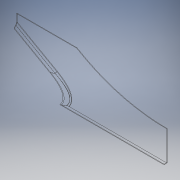
# Autodesk Inventor part: endplate
Saved by Autodesk Inventor 2018.2 (Build 222227000, 227)
## iProperties
Created: 2018-02-26
Part Number: endplate
Material: GFRC
Document SubType Name: Modeling
Designer: ku_sk
Density: 1.7 g/cm^3
Appearance: フラット - 研磨 グレー
Author: ku_sk
Autodesk Inventor part; units mm, degrees
ref_plane "YZ Plane" through (0, 0, 0) normal (1, 0, 0) x (0, 1, 0)
ref_plane "XZ Plane" through (0, 0, 0) normal (0, 1, 0) x (-1, 0, 0)
sketch "スケッチ1" plane through (0, 0, 0) normal (0, 1, 0) x (-1, 0, 0)
  line L0 (-250, 91.5) -> (250, 91.5)
  line L1 (250, 91.5) -> (250, -91.5)
  line L2 (250, -91.5) -> (-250, -91.5)
  line L3 (-250, -91.5) -> (-250, 91.5)
  line L4 (-250, 91.5) -> (250, -91.5) construction
  line L5 (250, 91.5) -> (-250, -91.5) construction
  point P0 (0, 0)
  dimension "d0" = 500
  dimension "d1" = 183
  constraints: 12 end point, 2 midpoint, 2 parallel, 1 horizontal, 1 perpendicular
  measures "d0" distance of L0.start L0.end
  measures "d1" distance of L0.end L1.end
extrude "押し出し1" add sketch "スケッチ1" along normal mid plane 10
ref_plane "作業平面1" through (250, 5, -91.5) normal (-0.8660254, -0.5, 0) x (0, 0, -1)
sketch "スケッチ2" plane through (250, 5, -91.5) normal (-0.8660254, -0.5, 0) x (0, 0, -1)
  ellipse E0 centre (-25, -530) end of major axis (-25, -900) minor radius 150
  line L0 (0, -250) -> (-183, -250) projected
  line L1 (0, 0) -> (0, -250) projected
  line L2 (-152.5782, -250) -> (-123.0545, -250)
  line L3 (-152.5782, -250) -> (-75.7791, -181.8461)
  point P0 (-91.5, -120.6699)
  dimension "d8" = 370
  dimension "d10" = 150
  dimension "d7" = 280
  dimension "d9" = 25
  constraints: 4 end point, 1 collinear, 1 horizontal, 1 point on line, 5 other
  measures "d7" distance from line of point (-25, -530) L0
  measures "d9" distance from line of L1 point (-25, -530)
extrude "押し出し2" cut sketch "スケッチ2" along normal through all
fillet "フィレット1" radius 10 1 edges at (-76.5294, 5, -46.6177)
shell "シェル1" thickness 2 removed faces 4 at (136.8712, -5, -18.4331) at (-250, -1.6667, 69.7349) at (-83.3333, 1.6667, 91.5) at (250, 1.6667, -30.5)
sketch "スケッチ3" plane through (0, 5, 0) normal (0, 1, 0) x (1, 0, 0)
  arc A0 (250, -8.5) -> (-50, -91.5) centre (250, -592.1687) ccw
  line L0 (250, -91.5) -> (250, 91.5) projected
  line L1 (-250, -91.5) -> (250, -91.5) projected
  line L2 (250, 91.5) -> (-76.2245, 91.5) projected
  line L3 (-250, -66.3852) -> (-250, -91.5) projected
  point P0 (0, 0)
  point P1 (-250, -29.9987)
  point P2 (-250, -57.7359)
  dimension "d13" = 100
  dimension "d14" = 200
  constraints: 2 point on circle, 2 point on line, 1 centre point, 1 line through centre
  measures "d13" distance from line of L2 A0.start
  measures "d14" distance from line of L3 A0.end
extrude "押し出し3" cut sketch "スケッチ3" against normal through all
